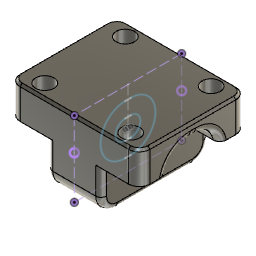
x_carriage_pivot_block (Autodesk Fusion 360 design; units mm, degrees)
Autodesk Fusion 360 part; units mm, degrees
sketch "Sketch1" plane through (0, 0, 0) normal (0, 0, 1) x (1, 0, 0) in component "x_carriage_pivot_block"
  line L0 (12.1, 10) -> (-12.1, 10)
  line L1 (-12.1, 10) -> (-12.1, -10)
  line L2 (-12.1, -10) -> (12.1, -10)
  line L3 (12.1, -10) -> (12.1, 10)
  line L4 (12.1, 10) -> (-12.1, -10) construction
  line L5 (-12.1, 10) -> (12.1, -10) construction
  dimension "d1" = 24.2
  dimension "d2" = 20
  constraint horizontal L0
  constraint perpendicular L0 L1
  constraint parallel L0 L2
  constraint parallel L1 L3
  constraint coincident L4 origin
  constraint coincident L5 origin
  measures "d1" distance of L1.end L2.end
  measures "d2" distance of L0.end L1.end
extrude "Extrude1" add sketch "Sketch1" along normal blind 6 in component "x_carriage_pivot_block"
sketch "Sketch2" plane through (0, 0, 0) normal (0, 0, -1) x (1, 0, 0) in component "x_carriage_pivot_block"
  line L0 (12.1, -10) -> (12.1, 10)
  line L1 (12.1, 10) -> (-12.1, 10)
  line L2 (-12.1, 10) -> (-12.1, -10)
  line L3 (-12.1, -10) -> (12.1, -10)
  line L4 (5, 10) -> (-5, 10)
  line L5 (-5, 10) -> (-5, -10)
  line L6 (-5, -10) -> (5, -10)
  line L7 (5, -10) -> (5, 10)
  line L8 (5, 10) -> (-5, -10) construction
  line L9 (-5, 10) -> (5, -10) construction
  dimension "d5" = 10
  dimension "d6" = 20
  constraint horizontal L4
  constraint perpendicular L4 L5
  constraint parallel L4 L6
  constraint parallel L5 L7
  constraint coincident L8 origin
  constraint coincident L9 origin
  measures "d5" distance of L5.end L6.end
  measures "d6" distance of L4.end L5.end
extrude "Extrude2" add sketch "Sketch2" along normal blind 8 contours L1 L3 L4 L5 L6 L7 in component "x_carriage_pivot_block"
sketch "Sketch3" plane through (0, 0, 0) normal (1, 0, 0) x (0, 1, 0) in component "x_carriage_pivot_block"
  line L0 (10, 0) -> (10, 6) construction
  line L1 (10, 6) -> (-10, 6) construction
  line L2 (-10, 6) -> (-10, 0) construction
  line L3 (-10, 0) -> (-10, -8) construction
  line L4 (-10, -8) -> (10, -8) construction
  line L5 (10, -8) -> (10, 0) construction
  line L6 (-0.5, -2.8) -> (0.5, -2.8)
  arc A0 (0.5, -2.8) -> (0.5, 0.8) centre (0.5, -1) ccw
  line L7 (0.5, 0.8) -> (-0.5, 0.8)
  arc A1 (-0.5, 0.8) -> (-0.5, -2.8) centre (-0.5, -1) ccw
  line L8 (-0.5, -1) -> (0.5, -1) construction
  line L9 (0, 6) -> (0, -8) construction
  line L10 (-0.5, -5.61) -> (0.5, -5.61)
  arc A2 (0.5, -5.61) -> (0.5, 3.61) centre (0.5, -1) ccw
  line L11 (0.5, 3.61) -> (-0.5, 3.61)
  arc A3 (-0.5, 3.61) -> (-0.5, -5.61) centre (-0.5, -1) ccw
  line L12 (-0.5, -1) -> (0.5, -1) construction
  point P0 (0, -1)
  dimension "d9" = 3.6
  dimension "d11" = 1
  dimension "d12" = 9.22
  constraint tangent L6 A0
  constraint tangent A0 L7
  constraint parallel L6 L7
  constraint tangent L7 A1
  constraint tangent L6 A1
  constraint parallel L1 L8
  constraint midpoint L1 L9.start
  constraint midpoint L4 L9.end
  constraint midpoint L9 P0
  constraint coincident L8 P0
  constraint tangent L10 A2
  constraint tangent A2 L11
  constraint parallel L10 L11
  constraint tangent L11 A3
  constraint tangent L10 A3
  constraint coincident A0.centre L8.end
  constraint perpendicular L9 L12
  constraint coincident A1.centre L8.start
  measures "d9" diameter of A0
  measures "d11" distance of A1.centre A0.centre
  measures "d12" diameter of A2
extrude "Extrude3" cut sketch "Sketch3" along normal through all and the other way through all contours L6 A0 L7 A1 in component "x_carriage_pivot_block"
extrude "Extrude4" cut sketch "Sketch3" along normal through all from surface at 5 in component "x_carriage_pivot_block"
extrude "Extrude5" cut sketch "Sketch3" against normal through all from surface at -5 in component "x_carriage_pivot_block"
sketch "Sketch4" plane through (0, 0, 6) normal (0, 0, 1) x (-1, 0, 0) in component "x_carriage_pivot_block"
  line L0 (-12.1, 10) -> (-12.1, -10)
  line L1 (-12.1, -10) -> (12.1, -10)
  line L2 (12.1, -10) -> (12.1, 10)
  line L3 (12.1, 10) -> (-12.1, 10)
  circle A0 centre (8, -7.5) radius 1.7
  line L4 (0, 0) -> (0, -13) construction
  line L5 (0, 0) -> (-15, 0) construction
  circle A1 centre (-8, -7.5) radius 1.7
  circle A2 centre (8, 7.5) radius 1.7
  circle A3 centre (-8, 7.5) radius 1.7
  dimension "d19" = 3.4
  dimension "d20" = 16
  dimension "d21" = 15
  constraint coincident L4.start L5.start
  constraint vertical L4
  constraint perpendicular L0 L5
  constraint symmetric A0 L4 A1
  constraint symmetric A0 L5 A2
  constraint symmetric L5 A1 A3
  measures "d19" diameter of A0
  measures "d20" distance of A0.centre A1.centre
  measures "d21" distance of A1.centre A3.centre
extrude "Extrude6" cut sketch "Sketch4" against normal through all contours A0 | A1 | A2 | A3 in component "x_carriage_pivot_block"
fillet "Fillet1" radius 3 2 edges at (0, -10, -8) (0, 10, -8) in component "x_carriage_pivot_block"
fillet "Fillet2" radius 1 10 edges at (-5, 10, -2.5) (-5, 9.1213, -7.1213) (-5, 0, -8) (-5, -9.1213, -7.1213) (-5, -10, -2.5) (5, 10, -2.5) (5, 9.1213, -7.1213) (5, 0, -8) (5, -9.1213, -7.1213) (5, -10, -2.5) in component "x_carriage_pivot_block"
fillet "Fillet3" radius 1.2 6 edges at (-12.1, 3.3846, 2.596) (-12.1, 0, 3.61) (-12.1, -3.3846, 2.596) (12.1, -3.3846, 2.596) (12.1, 0, 3.61) (12.1, 3.3846, 2.596) in component "x_carriage_pivot_block"
fillet "Fillet4" radius 0.8 6 edges at (-5, 3.3846, 2.596) (-5, 0, 3.61) (-5, -3.3846, 2.596) (5, -3.3846, 2.596) (5, 0, 3.61) (5, 3.3846, 2.596) in component "x_carriage_pivot_block"
fillet "Fillet5" radius 2 4 edges at (-12.1, 10, 3) (-12.1, -10, 3) (12.1, -10, 3) (12.1, 10, 3) in component "x_carriage_pivot_block"
chamfer "Chamfer1" distance 0.4 angle 45 8 edges at (12.1, 0, 6) (11.5142, 9.4142, 6) (0, 10, 6) (-11.5142, 9.4142, 6) (-12.1, 0, 6) (-11.5142, -9.4142, 6) (0, -10, 6) (11.5142, -9.4142, 6) in component "x_carriage_pivot_block"
component "x_carriage_pivot_block" placed x (1, 0, 0) y (0, 1, 0) z (0, 0, 1) at (0, 0, 0)
equation "pivot_movement = 1 mm"
equation "d11 = pivot_movement"
equation "d12 = ( 4.61 * 2 ) * 1 mm"
equation "d19 = ( 1.7 * 2 ) * 1 mm"
equation "d33 = chamfer"
equation "chamfer = 0.4 mm"
